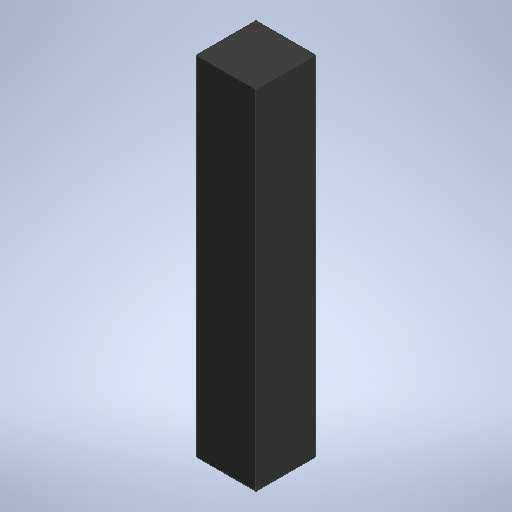
# Autodesk Inventor part: CableFemale
Saved by Autodesk Inventor 2025.1 (Build 291241020, 241B)
## iProperties
Created: 2024-09-01
Part Number: CableFemale
Material: Generic
Document SubType Name: Modeling
Designer: andre
Density: 1 g/cm^3
Appearance: Default
Author: andre
Autodesk Inventor part; units mm, degrees
ref_plane "YZ Plane" through (0, 0, 0) normal (1, 0, 0) x (0, 1, 0)
ref_plane "XZ Plane" through (0, 0, 0) normal (0, 1, 0) x (-1, 0, 0)
ref_plane "XY Plane" through (0, 0, 0) normal (0, 0, 1) x (1, 0, 0)
sketch "Sketch1" plane through (0, 0, 0) normal (0, 1, 0) x (-1, 0, 0)
  line L0 (0, 0) -> (2.4, 0)
  line L1 (2.4, 0) -> (2.4, -2.4)
  line L2 (2.4, -2.4) -> (0, -2.4)
  line L3 (0, -2.4) -> (0, 0)
  line L4 (1.595, -1.595) -> (0.805, -1.595)
  line L5 (0.805, -1.595) -> (0.805, -0.805)
  line L6 (0.805, -0.805) -> (1.595, -0.805)
  line L7 (1.595, -0.805) -> (1.595, -1.595)
  point P0 (1.2, -0.805)
  point P1 (1.2, 0)
  point P2 (1.595, -1.2)
  point P3 (2.4, -1.2)
  dimension "d0" = 2.4
  dimension "d1" = 2.4
  dimension "d2" = 0.79
  dimension "d3" = 0.79
  constraints: 16 end point, 4 midpoint, 4 parallel, 2 horizontal, 2 perpendicular, 1 horizontal alignment, 1 vertical alignment
  measures "d0" distance of L1.end L2.end
  measures "d1" distance of L0.end L1.end
  measures "d2" distance of L5.end L6.end
  measures "d3" distance of L4.end L5.end
extrude "Extrusion1" add sketch "Sketch1" along normal blind 14
sketch "Sketch2" plane through (0, 14, 0) normal (0, 1, 0) x (1, 0, 0)
  line L0 (-1.595, 0.805) -> (-1.595, 1.595) projected
  line L1 (0, 2.4) -> (-2.4, 2.4) projected
  line L2 (-2.4, 2.4) -> (-2.4, 0) projected
  line L3 (-2.4, 0) -> (0, 0) projected
  line L4 (0, 0) -> (0, 2.4) projected
  line L5 (-1.595, 1.595) -> (-0.805, 1.595) projected
  line L6 (-0.805, 1.595) -> (-0.805, 0.805) projected
  line L7 (-0.805, 0.805) -> (-1.595, 0.805) projected
  line L8 (-1.595, 0.805) -> (-1.595, 1.595) projected
extrude "Extrusion2" add sketch "Sketch2" against normal blind 2 contours L0 L5 L6 L7
body "Solid1"
